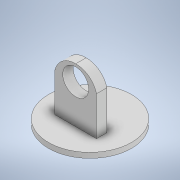
# Autodesk Inventor part: Base Top
Saved by Autodesk Inventor 2022 (Build 260153000, 153)
## iProperties
Created: 2022-01-28
Part Number: Base Top
Material: Generic
Document SubType Name: Modeling
Designer: Alexa
Density: 1 g/cm^3
Appearance: Default
Author: Alexa
Autodesk Inventor part; units mm, degrees
ref_plane "YZ Plane" through (0, 0, 0) normal (1, 0, 0) x (0, 1, 0)
ref_plane "XZ Plane" through (0, 0, 0) normal (0, 1, 0) x (-1, 0, 0)
ref_plane "XY Plane" through (0, 0, 0) normal (0, 0, 1) x (1, 0, 0)
sketch "Sketch1" plane through (0, 0, 0) normal (0, 1, 0) x (-1, 0, 0)
  circle A0 centre (0, 0) radius 80
  circle A1 centre (0, 0) radius 7.5
  dimension "d0" = 160
  dimension "d1" = 15
  constraints: 2 centre point, 2 coincident
  measures "d0" diameter of A0
  measures "d1" diameter of A1
extrude "Extrusion1" add sketch "Sketch1" along normal blind 10
sketch "Sketch2" plane through (0, 10, 0) normal (0, 1, 0) x (1, 0, 0)
  circle A0 centre (0, 0) radius 7.5 projected
  line L0 (0, -7.5) -> (-40, -7.5)
  line L1 (-40, -7.5) -> (-40, -27.5)
  line L2 (-40, -27.5) -> (0, -27.5)
  line L3 (0, -27.5) -> (0, -7.5)
  line L4 (0, -27.5) -> (40, -27.5)
  line L5 (40, -27.5) -> (40, -7.5)
  line L6 (40, -7.5) -> (0, -7.5)
  line L7 (0, -7.5) -> (0, -27.5)
  dimension "d4" = 40
  dimension "d5" = 20
  dimension "d6" = 40
  constraints: 16 end point, 4 parallel, 2 horizontal, 2 perpendicular, 1 vertical alignment, 1 other
  measures "d4" distance of L2.end L1.end
  measures "d5" distance between parallel lines of L0 L2
  measures "d6" distance of L6.end L5.end
extrude "Extrusion2" add sketch "Sketch2" along normal blind 150 contours L6 L5 L4 L3 | L3 L2 L1 L0
sketch "Sketch3" plane through (-40, 10, 27.5) normal (0, 0, 1) x (1, 0, 0)
  circle A0 centre (40, 75) radius 25
  line L0 (0, 150) -> (80, 150) projected
  line L1 (80, 0) -> (80, 150) projected
  line L2 (0, 150) -> (80, 150)
  line L3 (80, 150) -> (80, 105)
  line L4 (80, 105) -> (0, 105)
  line L5 (0, 105) -> (0, 150)
  line L6 (0, 0) -> (0, 150) projected
  arc A1 (40, 105) -> (0, 75) centre (38.735, 65.02) ccw
  arc A2 (80, 75) -> (40, 105) centre (41.265, 65.02) ccw
  point P0 (40, -10)
  dimension "d9" = 50
  dimension "d10" = 45
  dimension "d11" = 40
  dimension "d12" = 40
  constraints: 8 end point, 4 point on circle, 3 centre point, 3 midpoint, 2 parallel, 1 horizontal, 1 perpendicular, 1 point on line
  measures "d9" diameter of A0
  measures "d10" distance of L2.end L3.end
  measures "d11" radius of A1
  measures "d12" radius of A2
extrude "Extrusion3" cut sketch "Sketch3" against normal blind 21.45 contours A0 | L0 L1 L4 A2 A1 L5 | L4 A1 L6 | L1 A2 L4
sketch "Sketch4" plane through (-40, 10, 27.5) normal (0, 0, 1) x (1, 0, 0)
  point P0 (40, -10)
body "Solid1"
